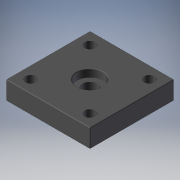
# Autodesk Inventor part: ball-holder-to-post-adapter
Saved by Autodesk Inventor 2019 (Build 230136000, 136)
## iProperties
Created: 2019-04-17
Part Number: ball-holder-to-post-adapter
Material: ABS Plastic
Document SubType Name: Modeling
Designer: Wilson Lab
Density: 1.06 g/cm^3
Appearance: Smooth - White
Author: Wilson Lab
Autodesk Inventor part; units mm, degrees
ref_plane "YZ Plane" through (0, 0, 0) normal (1, 0, 0) x (0, 1, 0)
ref_plane "XZ Plane" through (0, 0, 0) normal (0, 1, 0) x (-1, 0, 0)
ref_plane "XY Plane" through (0, 0, 0) normal (0, 0, 1) x (1, 0, 0)
sketch "Sketch1" plane through (0, 0, 0) normal (0, 1, 0) x (-1, 0, 0)
  line L0 (-18, 18) -> (18, 18)
  line L1 (18, 18) -> (18, -18)
  line L2 (18, -18) -> (-18, -18)
  line L3 (-18, -18) -> (-18, 18)
  line L4 (-18, 18) -> (18, -18) construction
  line L5 (18, 18) -> (-18, -18) construction
  point P0 (0, 0)
  dimension "d0" = 36
  dimension "d1" = 36
  constraints: 12 end point, 2 midpoint, 2 parallel, 1 horizontal, 1 perpendicular
  measures "d0" distance between parallel lines of L3 L1
  measures "d1" distance of L0.end L1.end
extrude "Extrusion1" add sketch "Sketch1" along normal blind 7.9375
sketch "Sketch3" plane through (0, 7.9375, 0) normal (0, 1, 0) x (1, 0, 0)
  line L0 (-12.7, -12.7) -> (12.7, -12.7) construction
  line L1 (12.7, -12.7) -> (12.7, 12.7) construction
  line L2 (12.7, 12.7) -> (-12.7, 12.7) construction
  line L3 (-12.7, 12.7) -> (-12.7, -12.7) construction
  line L4 (-12.7, -12.7) -> (12.7, 12.7) construction
  line L5 (12.7, -12.7) -> (-12.7, 12.7) construction
  point P0 (0, 0)
  dimension "d11" = 25.4
  constraints: 12 end point, 4 coincident, 2 midpoint, 2 parallel, 2 perpendicular, 1 horizontal
  measures "d11" distance of L1.end L2.end
hole "Hole2" at (-12.7, 7.9375, -12.7) at (12.7, 7.9375, -12.7) at (-12.7, 7.9375, 12.7) at (12.7, 7.9375, 12.7) direction (0, -1, 0) diameter 4.496 depth 12.3 tip angle 118 clearance for "Flat Head Machine Screw (82)" size "#8" standard "Ansi Unified Screw Threads"
sketch "Sketch2" plane through (0, 7.9375, 0) normal (0, 1, 0) x (1, 0, 0)
  point P0 (0, 0)
  point P1 (0, 0)
  constraints: 1 coincident
hole "Hole1" at (0, 7.9375, 0) direction (0, -1, 0) diameter 6.528 end through all counterbore diameter 11.113 counterbore depth 3.25 clearance for "Socket Head Cap Screw" size "1/4" standard "Ansi Unified Screw Threads"
fillet "Fillet1" radius 0.25 12 edges at (-18, 3.9688, 18) (0, 0, 18) (18, 3.9688, 18) (0, 7.9375, 18) (18, 7.9375, 0) (0, 7.9375, -18) (-18, 7.9375, 0) (18, 0, 0) (18, 3.9688, -18) (-18, 0, 0) (0, 0, -18) (-18, 3.9688, -18)
fillet "Fillet2" radius 0.25 1 edges at (0, 7.9375, -5.5565)
sketch "Sketch4" plane through (0, 0, 0) normal (0, -1, 0) x (1, 0, 0)
  circle A0 centre (0, 0) radius 12.687
  dimension "d21" = 25.374
  constraints: 1 centre point, 1 coincident
  measures "d21" diameter of A0
extrude "Extrusion2" cut sketch "Sketch4" against normal blind 1.5875
body "Solid1"
